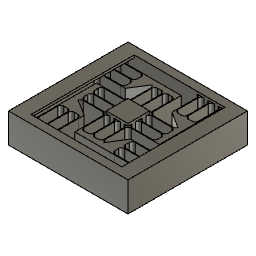
smaller mill draft (Autodesk Fusion 360 design; units mm, degrees)
part number: Configuration 5
Autodesk Fusion 360 part; units mm, degrees
(part 1 of 2)
sketch "Sketch2" plane through (0, 0, 0) normal (0, 0, 1) x (1, 0, 0) in component "xy"
  line L0 (-95, 0) -> (-95, -95)
  line L1 (-95, -95) -> (0, -95)
  line L2 (0, -20) -> (0, 0)
  line L3 (-38, -95) -> (-38, -47)
  line L4 (-78, -95) -> (-78, -47)
  line L5 (0, 0) -> (-20, 0)
  line L6 (-20, 0) -> (-20, -20)
  line L7 (-20, -20) -> (0, -20)
  line L8 (0, -20) -> (0, 0)
  line L9 (-20, -20) -> (-68, -20)
  line L10 (-110, 0) -> (-110, -110)
  line L11 (-110, -110) -> (0, -110)
  line L12 (-68, -24) -> (-38, -43)
  line L13 (-38, -43) -> (-38, -47)
  line L14 (-38, -47) -> (-78, -47)
  line L15 (0, -95) -> (0, -110)
  line L16 (-95, 0) -> (-110, 0)
  line L17 (-95, 0) -> (-110, 0) construction
  line L18 (0, -110) -> (0, -95) construction
  line L19 (0, -20) -> (0, 0) construction
  line L20 (0, 0) -> (-110, 0) construction
  line L21 (-110, 0) -> (-110, -110) construction
  line L22 (-110, -110) -> (0, -110) construction
  line L23 (0, -110) -> (0, 0) construction
  line L24 (-58, -47) -> (-58, -95) construction
  line L25 (-58.9, -71) -> (-57.1, -71) construction
  line L26 (-58.9, -47) -> (-58.9, -95)
  line L27 (-57.1, -95) -> (-57.1, -47)
  line L28 (-39.8, -95) -> (-39.8, -47)
  line L29 (-76.2, -95) -> (-76.2, -47)
  line L30 (-20, -18.2) -> (-68, -18.2)
  line L31 (0, 0) -> (-20, 0)
  line L32 (-190, 0) -> (-210, 0) construction
  line L33 (-20, 0.9) -> (-68, 0.9)
  line L34 (-20, -0.9) -> (-68, -0.9)
  line L35 (-44, -0.9) -> (-44, 0.9) construction
  line L36 (-20, 0.9) -> (-20, 0)
  line L37 (-20, 18.2) -> (-68, 18.2)
  line L38 (-20, 20) -> (-68, 20)
  line L39 (-78, -47) -> (-78, 20)
  line L40 (-78, 20) -> (-68, 20)
  line L41 (-68, 20) -> (-68, -24)
  line L42 (-20, 18.2) -> (-20, 20)
  line L43 (-20, 20) -> (-20, -18.2)
  line L44 (-20, -20) -> (20, -20)
  line L45 (20, -20) -> (20, 20)
  line L46 (20, 20) -> (-20, 20)
  line L47 (-20, 20) -> (-20, -20)
  line L48 (-20, -20) -> (20, 20) construction
  line L49 (20, -20) -> (-20, 20) construction
  point P0 (-44, 0)
  dimension "d47" = 40
  dimension "d48" = 17
  dimension "d52" = 15
  dimension "d56" = 4
  dimension "d57" = 110
  dimension "d60" = -1.8
  dimension "d64" = 40
  dimension "d86" = 10
  dimension "d117" = 4
  constraint vertical L0
  constraint horizontal L1
  constraint vertical L2
  constraint coincident L2.end L5.start
  constraint coincident L1 L3.start
  constraint perpendicular L1 L3
  constraint coincident L1 L4.start
  constraint perpendicular L1 L4
  constraint equal L3 L4
  constraint horizontal L5
  constraint vertical L6
  constraint horizontal L7
  constraint vertical L8
  constraint equal L6 L7
  constraint perpendicular L6 L9
  constraint equal L4 L9
  constraint horizontal L31
  constraint vertical L10
  constraint horizontal L11
  constraint vertical L18
  constraint equal L10 L11
  constraint vertical L13
  constraint horizontal L14
  constraint coincident L4.end L14.end
  constraint coincident L3.end L13.end
  constraint collinear L17 L31
  constraint collinear L18 L19
  constraint horizontal L20
  constraint vertical L21
  constraint horizontal L22
  constraint vertical L23
  constraint equal L0 L1
  constraint midpoint L14 L24.start
  constraint coincident L1 L24.end
  constraint perpendicular L1 L24
  constraint perpendicular L24 L25
  constraint midpoint L24 L25
  constraint coincident L14 L26.start
  constraint coincident L1 L26.end
  constraint perpendicular L1 L26
  constraint coincident L1 L27.start
  constraint coincident L14 L27.end
  constraint perpendicular L14 L27
  constraint coincident L25.start L26
  constraint coincident L25.end L27
  constraint horizontal L33
  constraint parallel L33 L34
  constraint midpoint L34 L35.start
  constraint coincident L33 L35.end
  constraint perpendicular L33 L35
  constraint midpoint L33 L35.end
  constraint equal L33 L34
  constraint coincident L6 L34.start
  constraint midpoint L35 P0
  constraint coincident L20 P0
  constraint symmetric L6.end L20 L38.start
  constraint symmetric L9.end L20 L38.end
  constraint symmetric L20 L30.start L37.start
  constraint symmetric L20 L30.end L37.end
  constraint vertical L39
  constraint horizontal L40
  constraint vertical L41
  constraint coincident L38.end L40.end
  constraint perpendicular L38 L42
  constraint horizontal L44
  constraint perpendicular L44 L45
  constraint parallel L44 L46
  constraint parallel L45 L47
  constraint coincident L48 L2.end
  constraint coincident L49 L2.end
  constraint coincident L33.end L41
  measures "d47" distance of L3 L4
  measures "d48" distance of L0.end L4
  measures "d52" distance of L0 L10
  measures "d56" distance of L9.end L12.start
  measures "d57" distance of L10.start L10.end
  measures "d86" distance of L12.start L39
  measures "d117" distance of L12.end L3.end
extrude "Extrude3" add sketch "Sketch2" along normal mid plane 67.5 contours L2 L5 L8 L31 L36 L42 L43 L44 L45 L46 L47 | L2 L5 L6 L7 L8 L31 L43 L44 L47 makes body 1 in component "xy"
extrude "Extrude2" add sketch "Sketch2" along normal mid plane 67.5 separate body contours L0 L1 L10 L11 L15 L16 | L1 L4 L14 L29 | L12 L13 L14 L39 L40 L41 | L1 L14 L26 L27 | L37 L38 L41 L42 L43 L47 | L1 L3 L14 L28 | L6 L33 L34 L36 L41 L43 L47 | L6 L9 L30 L41 L47 makes body 2 in component "xy"
combine "Combine2" operation add target body 1 tool bodies 2 in component "xy"
fillet "Fillet2" radius 5.558 19 edges at (-20, -18.2, 0) (-20, 0.9, 0) (-20, 18.2, 0) (-20, -0.9, 0) (-68, -18.2, 0) (-68, -20, 0) (-68, 0.9, 0) (-68, -0.9, 0) (-68, 18.2, 0) (-38, -95, 0) (-57.1, -95, 0) (-76.2, -95, 0) (-78, -95, 0) (-39.8, -95, 0) (-58.9, -95, 0) (-76.2, -47, 0) (-57.1, -47, 0) (-39.8, -47, 0) (-58.9, -47, 0) on bodies 1 in component "xy"
pattern_circular "C-Pattern3" count 4 over 360 about axis through (0, 0, 1.75) along (0, 0, 1) of bodies 1 makes body 3 at (110, -73.3333, 11.25) makes body 4 at (73.3333, 110, 11.25) makes body 5 at (-110, 73.3333, 11.25) in component "xy"
combine "Combine3" operation add target body 3 tool bodies 1 5 4 in component "xy"
fillet "Fillet4" radius 6.013 4 edges at (-20, 20, 0) (20, 20, 0) (20, -20, 0) (-20, -20, 0) on bodies 3 in component "xy"
sketch "Sketch3" plane through (0, 0, 33.75) normal (0, 0, 1) x (-1, 0, 0) in component "xy"
  line L0 (-110, -110) -> (110, -110)
  line L1 (110, -110) -> (110, 110)
  line L2 (110, 110) -> (-110, 110)
  line L3 (-110, 110) -> (-110, -110)
  line L4 (-95, -95) -> (-95, 32.442)
  arc A0 (-89.442, 38) -> (-95, 32.442) centre (-89.442, 32.442) ccw
  line L5 (-89.442, 38) -> (-43, 38)
  line L6 (-43, 38) -> (-24, 68)
  arc A1 (-20, 62.6648) -> (-24, 68) centre (-25.558, 62.6648) ccw
  line L7 (-20, 62.6648) -> (-20, 26.013)
  arc A2 (-26.013, 20) -> (-20, 26.013) centre (-26.013, 26.013) ccw
  line L8 (-26.013, 20) -> (-78, 20)
  line L9 (-78, 20) -> (-78, -89.442)
  arc A3 (-83.558, -95) -> (-78, -89.442) centre (-83.558, -89.442) ccw
  line L10 (-83.558, -95) -> (-95, -95)
  line L11 (-20, 12.642) -> (-20, 6.458)
  arc A4 (-25.558, 0.9) -> (-20, 6.458) centre (-25.558, 6.458) ccw
  line L12 (-25.558, 0.9) -> (-62.442, 0.9)
  arc A5 (-68, 6.458) -> (-62.442, 0.9) centre (-62.442, 6.458) ccw
  line L13 (-68, 6.458) -> (-68, 12.642)
  arc A6 (-62.442, 18.2) -> (-68, 12.642) centre (-62.442, 12.642) ccw
  line L14 (-62.442, 18.2) -> (-25.558, 18.2)
  arc A7 (-20, 12.642) -> (-25.558, 18.2) centre (-25.558, 12.642) ccw
  line L15 (-20, -6.458) -> (-20, -12.642)
  arc A8 (-25.558, -18.2) -> (-20, -12.642) centre (-25.558, -12.642) ccw
  line L16 (-25.558, -18.2) -> (-62.442, -18.2)
  arc A9 (-68, -12.642) -> (-62.442, -18.2) centre (-62.442, -12.642) ccw
  line L17 (-68, -12.642) -> (-68, -6.458)
  arc A10 (-62.442, -0.9) -> (-68, -6.458) centre (-62.442, -6.458) ccw
  line L18 (-62.442, -0.9) -> (-25.558, -0.9)
  arc A11 (-20, -6.458) -> (-25.558, -0.9) centre (-25.558, -6.458) ccw
  line L19 (-45.358, -95) -> (-51.542, -95)
  arc A12 (-57.1, -89.442) -> (-51.542, -95) centre (-51.542, -89.442) ccw
  line L20 (-57.1, -89.442) -> (-57.1, -52.558)
  arc A13 (-51.542, -47) -> (-57.1, -52.558) centre (-51.542, -52.558) ccw
  line L21 (-51.542, -47) -> (-45.358, -47)
  arc A14 (-39.8, -52.558) -> (-45.358, -47) centre (-45.358, -52.558) ccw
  line L22 (-39.8, -52.558) -> (-39.8, -89.442)
  arc A15 (-45.358, -95) -> (-39.8, -89.442) centre (-45.358, -89.442) ccw
  line L23 (-70.642, -47) -> (-64.458, -47)
  arc A16 (-58.9, -52.558) -> (-64.458, -47) centre (-64.458, -52.558) ccw
  line L24 (-58.9, -52.558) -> (-58.9, -89.442)
  arc A17 (-64.458, -95) -> (-58.9, -89.442) centre (-64.458, -89.442) ccw
  line L25 (-64.458, -95) -> (-70.642, -95)
  arc A18 (-76.2, -89.442) -> (-70.642, -95) centre (-70.642, -89.442) ccw
  line L26 (-76.2, -89.442) -> (-76.2, -52.558)
  arc A19 (-70.642, -47) -> (-76.2, -52.558) centre (-70.642, -52.558) ccw
  arc A20 (-18.2, 25.558) -> (-12.642, 20) centre (-12.642, 25.558) ccw
  line L27 (-18.2, 25.558) -> (-18.2, 62.442)
  arc A21 (-12.642, 68) -> (-18.2, 62.442) centre (-12.642, 62.442) ccw
  line L28 (-12.642, 68) -> (-6.458, 68)
  arc A22 (-0.9, 62.442) -> (-6.458, 68) centre (-6.458, 62.442) ccw
  line L29 (-0.9, 62.442) -> (-0.9, 25.558)
  arc A23 (-6.458, 20) -> (-0.9, 25.558) centre (-6.458, 25.558) ccw
  line L30 (-6.458, 20) -> (-12.642, 20)
  arc A24 (0.9, 25.558) -> (6.458, 20) centre (6.458, 25.558) ccw
  line L31 (0.9, 25.558) -> (0.9, 62.442)
  arc A25 (6.458, 68) -> (0.9, 62.442) centre (6.458, 62.442) ccw
  line L32 (6.458, 68) -> (12.642, 68)
  arc A26 (18.2, 62.442) -> (12.642, 68) centre (12.642, 62.442) ccw
  line L33 (18.2, 62.442) -> (18.2, 25.558)
  arc A27 (12.642, 20) -> (18.2, 25.558) centre (12.642, 25.558) ccw
  line L34 (12.642, 20) -> (6.458, 20)
  line L35 (20, 26.013) -> (20, 78)
  line L36 (20, 78) -> (-89.442, 78)
  arc A28 (-95, 83.558) -> (-89.442, 78) centre (-89.442, 83.558) ccw
  line L37 (-95, 83.558) -> (-95, 95)
  line L38 (-95, 95) -> (32.442, 95)
  arc A29 (38, 89.442) -> (32.442, 95) centre (32.442, 89.442) ccw
  line L39 (38, 89.442) -> (38, 43)
  line L40 (38, 43) -> (68, 24)
  arc A30 (62.6648, 20) -> (68, 24) centre (62.6648, 25.558) ccw
  line L41 (62.6648, 20) -> (26.013, 20)
  arc A31 (20, 26.013) -> (26.013, 20) centre (26.013, 26.013) ccw
  line L42 (95, -95) -> (-32.442, -95)
  arc A32 (-38, -89.442) -> (-32.442, -95) centre (-32.442, -89.442) ccw
  line L43 (-38, -89.442) -> (-38, -43)
  line L44 (-38, -43) -> (-68, -24)
  arc A33 (-62.6648, -20) -> (-68, -24) centre (-62.6648, -25.558) ccw
  line L45 (-62.6648, -20) -> (-26.013, -20)
  arc A34 (-20, -26.013) -> (-26.013, -20) centre (-26.013, -26.013) ccw
  line L46 (-20, -26.013) -> (-20, -78)
  line L47 (-20, -78) -> (89.442, -78)
  arc A35 (95, -83.558) -> (89.442, -78) centre (89.442, -83.558) ccw
  line L48 (95, -83.558) -> (95, -95)
  arc A36 (25.558, 18.2) -> (20, 12.642) centre (25.558, 12.642) ccw
  line L49 (25.558, 18.2) -> (62.442, 18.2)
  arc A37 (68, 12.642) -> (62.442, 18.2) centre (62.442, 12.642) ccw
  line L50 (68, 12.642) -> (68, 6.458)
  arc A38 (62.442, 0.9) -> (68, 6.458) centre (62.442, 6.458) ccw
  line L51 (62.442, 0.9) -> (25.558, 0.9)
  arc A39 (20, 6.458) -> (25.558, 0.9) centre (25.558, 6.458) ccw
  line L52 (20, 6.458) -> (20, 12.642)
  line L53 (-12.642, -20) -> (-6.458, -20)
  arc A40 (-0.9, -25.558) -> (-6.458, -20) centre (-6.458, -25.558) ccw
  line L54 (-0.9, -25.558) -> (-0.9, -62.442)
  arc A41 (-6.458, -68) -> (-0.9, -62.442) centre (-6.458, -62.442) ccw
  line L55 (-6.458, -68) -> (-12.642, -68)
  arc A42 (-18.2, -62.442) -> (-12.642, -68) centre (-12.642, -62.442) ccw
  line L56 (-18.2, -62.442) -> (-18.2, -25.558)
  arc A43 (-12.642, -20) -> (-18.2, -25.558) centre (-12.642, -25.558) ccw
  arc A44 (25.558, -0.9) -> (20, -6.458) centre (25.558, -6.458) ccw
  line L57 (25.558, -0.9) -> (62.442, -0.9)
  arc A45 (68, -6.458) -> (62.442, -0.9) centre (62.442, -6.458) ccw
  line L58 (68, -6.458) -> (68, -12.642)
  arc A46 (62.442, -18.2) -> (68, -12.642) centre (62.442, -12.642) ccw
  line L59 (62.442, -18.2) -> (25.558, -18.2)
  arc A47 (20, -12.642) -> (25.558, -18.2) centre (25.558, -12.642) ccw
  line L60 (20, -12.642) -> (20, -6.458)
  line L61 (6.458, -20) -> (12.642, -20)
  arc A48 (18.2, -25.558) -> (12.642, -20) centre (12.642, -25.558) ccw
  line L62 (18.2, -25.558) -> (18.2, -62.442)
  arc A49 (12.642, -68) -> (18.2, -62.442) centre (12.642, -62.442) ccw
  line L63 (12.642, -68) -> (6.458, -68)
  arc A50 (0.9, -62.442) -> (6.458, -68) centre (6.458, -62.442) ccw
  line L64 (0.9, -62.442) -> (0.9, -25.558)
  arc A51 (6.458, -20) -> (0.9, -25.558) centre (6.458, -25.558) ccw
  line L65 (-95, 45.358) -> (-95, 51.542)
  arc A52 (-89.442, 57.1) -> (-95, 51.542) centre (-89.442, 51.542) ccw
  line L66 (-89.442, 57.1) -> (-52.558, 57.1)
  arc A53 (-47, 51.542) -> (-52.558, 57.1) centre (-52.558, 51.542) ccw
  line L67 (-47, 51.542) -> (-47, 45.358)
  arc A54 (-52.558, 39.8) -> (-47, 45.358) centre (-52.558, 45.358) ccw
  line L68 (-52.558, 39.8) -> (-89.442, 39.8)
  arc A55 (-95, 45.358) -> (-89.442, 39.8) centre (-89.442, 45.358) ccw
  line L69 (-47, 70.642) -> (-47, 64.458)
  arc A56 (-52.558, 58.9) -> (-47, 64.458) centre (-52.558, 64.458) ccw
  line L70 (-52.558, 58.9) -> (-89.442, 58.9)
  arc A57 (-95, 64.458) -> (-89.442, 58.9) centre (-89.442, 64.458) ccw
  line L71 (-95, 64.458) -> (-95, 70.642)
  arc A58 (-89.442, 76.2) -> (-95, 70.642) centre (-89.442, 70.642) ccw
  line L72 (-89.442, 76.2) -> (-52.558, 76.2)
  arc A59 (-47, 70.642) -> (-52.558, 76.2) centre (-52.558, 70.642) ccw
  line L73 (45.358, 95) -> (51.542, 95)
  arc A60 (57.1, 89.442) -> (51.542, 95) centre (51.542, 89.442) ccw
  line L74 (57.1, 89.442) -> (57.1, 52.558)
  arc A61 (51.542, 47) -> (57.1, 52.558) centre (51.542, 52.558) ccw
  line L75 (51.542, 47) -> (45.358, 47)
  arc A62 (39.8, 52.558) -> (45.358, 47) centre (45.358, 52.558) ccw
  line L76 (39.8, 52.558) -> (39.8, 89.442)
  arc A63 (45.358, 95) -> (39.8, 89.442) centre (45.358, 89.442) ccw
  line L77 (70.642, 47) -> (64.458, 47)
  arc A64 (58.9, 52.558) -> (64.458, 47) centre (64.458, 52.558) ccw
  line L78 (58.9, 52.558) -> (58.9, 89.442)
  arc A65 (64.458, 95) -> (58.9, 89.442) centre (64.458, 89.442) ccw
  line L79 (64.458, 95) -> (70.642, 95)
  arc A66 (76.2, 89.442) -> (70.642, 95) centre (70.642, 89.442) ccw
  line L80 (76.2, 89.442) -> (76.2, 52.558)
  arc A67 (70.642, 47) -> (76.2, 52.558) centre (70.642, 52.558) ccw
  line L81 (47, -70.642) -> (47, -64.458)
  arc A68 (52.558, -58.9) -> (47, -64.458) centre (52.558, -64.458) ccw
  line L82 (52.558, -58.9) -> (89.442, -58.9)
  arc A69 (95, -64.458) -> (89.442, -58.9) centre (89.442, -64.458) ccw
  line L83 (95, -64.458) -> (95, -70.642)
  arc A70 (89.442, -76.2) -> (95, -70.642) centre (89.442, -70.642) ccw
  line L84 (89.442, -76.2) -> (52.558, -76.2)
  arc A71 (47, -70.642) -> (52.558, -76.2) centre (52.558, -70.642) ccw
  line L85 (95, -45.358) -> (95, -51.542)
  arc A72 (89.442, -57.1) -> (95, -51.542) centre (89.442, -51.542) ccw
  line L86 (89.442, -57.1) -> (52.558, -57.1)
  arc A73 (47, -51.542) -> (52.558, -57.1) centre (52.558, -51.542) ccw
  line L87 (47, -51.542) -> (47, -45.358)
  arc A74 (52.558, -39.8) -> (47, -45.358) centre (52.558, -45.358) ccw
  line L88 (52.558, -39.8) -> (89.442, -39.8)
  arc A75 (95, -45.358) -> (89.442, -39.8) centre (89.442, -45.358) ccw
  line L89 (26.013, -20) -> (78, -20)
  line L90 (78, -20) -> (78, 89.442)
  arc A76 (83.558, 95) -> (78, 89.442) centre (83.558, 89.442) ccw
  line L91 (83.558, 95) -> (95, 95)
  line L92 (95, 95) -> (95, -32.442)
  arc A77 (89.442, -38) -> (95, -32.442) centre (89.442, -32.442) ccw
  line L93 (89.442, -38) -> (43, -38)
  line L94 (43, -38) -> (24, -68)
  arc A78 (20, -62.6648) -> (24, -68) centre (25.558, -62.6648) ccw
  line L95 (20, -62.6648) -> (20, -26.013)
  arc A79 (26.013, -20) -> (20, -26.013) centre (26.013, -26.013) ccw
  line L96 (-20, 20) -> (20, 20)
  line L97 (20, 20) -> (20, -20)
  line L98 (20, -20) -> (-20, -20)
  line L99 (-20, -20) -> (-20, 20)
  line L100 (-20, 20) -> (20, -20) construction
  line L101 (20, 20) -> (-20, -20) construction
  line L102 (-95, 95) -> (95, 95)
  line L103 (95, 95) -> (95, -95)
  line L104 (95, -95) -> (-95, -95)
  line L105 (-95, -95) -> (-95, 95)
  line L106 (-95, 95) -> (95, -95) construction
  line L107 (95, 95) -> (-95, -95) construction
  line L108 (-110, 110) -> (110, 110)
  line L109 (110, 110) -> (110, -110)
  line L110 (110, -110) -> (-110, -110)
  line L111 (-110, -110) -> (-110, 110)
  line L112 (-110, 110) -> (110, -110) construction
  line L113 (110, 110) -> (-110, -110) construction
  constraint horizontal L96
  constraint perpendicular L96 L97
  constraint parallel L96 L98
  constraint parallel L97 L99
  constraint coincident L100 origin
  constraint coincident L101 origin
  constraint horizontal L102
  constraint perpendicular L102 L103
  constraint parallel L102 L104
  constraint parallel L103 L105
  constraint coincident L106 origin
  constraint coincident L107 origin
  constraint coincident L37.end L38.start
  constraint horizontal L108
  constraint perpendicular L108 L109
  constraint parallel L108 L110
  constraint parallel L109 L111
  constraint coincident L112 origin
  constraint coincident L113 origin
  constraint coincident L2.end L3.start
extrude "Extrude4" add sketch "Sketch3" along normal blind 1 contours L0 L1 L2 L3 L108 L109 L110 L111 | L11 L15 L30 L34 L52 L53 L60 L61 L96 L97 L98 L99 bodies 3 in component "xy"
sketch "Sketch2 (1)" plane through (0, 0, 0) normal (0, 0, 1) x (1, 0, 0) in component "xy"
copy_body "Body->Comp1" bodies 3 removing the originals makes body 6 in component "main xy flex"
sketch "Sketch3 (2)" plane through (0, 0, 33.75) normal (0, 0, 1) x (-1, 0, 0)
  line L0 (20, 20) -> (20, 12.642)
  arc A0 (25.558, 18.2) -> (20, 12.642) centre (25.558, 12.642) ccw
  line L1 (25.558, 18.2) -> (62.442, 18.2)
  arc A1 (68, 12.642) -> (62.442, 18.2) centre (62.442, 12.642) ccw
  line L2 (68, 12.642) -> (68, 6.458)
  arc A2 (62.442, 0.9) -> (68, 6.458) centre (62.442, 6.458) ccw
  line L3 (62.442, 0.9) -> (25.558, 0.9)
  arc A3 (20, 6.458) -> (25.558, 0.9) centre (25.558, 6.458) ccw
  line L4 (20, 6.458) -> (20, -6.458)
  arc A4 (25.558, -0.9) -> (20, -6.458) centre (25.558, -6.458) ccw
  line L5 (25.558, -0.9) -> (62.442, -0.9)
  arc A5 (68, -6.458) -> (62.442, -0.9) centre (62.442, -6.458) ccw
  line L6 (68, -6.458) -> (68, -12.642)
  arc A6 (62.442, -18.2) -> (68, -12.642) centre (62.442, -12.642) ccw
  line L7 (62.442, -18.2) -> (25.558, -18.2)
  arc A7 (20, -12.642) -> (25.558, -18.2) centre (25.558, -12.642) ccw
  line L8 (20, -12.642) -> (20, -20)
  line L9 (20, -20) -> (12.642, -20)
  arc A8 (18.2, -25.558) -> (12.642, -20) centre (12.642, -25.558) ccw
  line L10 (18.2, -25.558) -> (18.2, -62.442)
  arc A9 (12.642, -68) -> (18.2, -62.442) centre (12.642, -62.442) ccw
  line L11 (12.642, -68) -> (6.458, -68)
  arc A10 (0.9, -62.442) -> (6.458, -68) centre (6.458, -62.442) ccw
  line L12 (0.9, -62.442) -> (0.9, -25.558)
  arc A11 (6.458, -20) -> (0.9, -25.558) centre (6.458, -25.558) ccw
  line L13 (6.458, -20) -> (-6.458, -20)
  arc A12 (-0.9, -25.558) -> (-6.458, -20) centre (-6.458, -25.558) ccw
  line L14 (-0.9, -25.558) -> (-0.9, -62.442)
  arc A13 (-6.458, -68) -> (-0.9, -62.442) centre (-6.458, -62.442) ccw
  line L15 (-6.458, -68) -> (-12.642, -68)
  arc A14 (-18.2, -62.442) -> (-12.642, -68) centre (-12.642, -62.442) ccw
  line L16 (-18.2, -62.442) -> (-18.2, -25.558)
  arc A15 (-12.642, -20) -> (-18.2, -25.558) centre (-12.642, -25.558) ccw
  line L17 (-12.642, -20) -> (-20, -20)
  line L18 (-20, -20) -> (-20, -12.642)
  arc A16 (-25.558, -18.2) -> (-20, -12.642) centre (-25.558, -12.642) ccw
  line L19 (-25.558, -18.2) -> (-62.442, -18.2)
  arc A17 (-68, -12.642) -> (-62.442, -18.2) centre (-62.442, -12.642) ccw
  line L20 (-68, -12.642) -> (-68, -6.458)
  arc A18 (-62.442, -0.9) -> (-68, -6.458) centre (-62.442, -6.458) ccw
  line L21 (-62.442, -0.9) -> (-25.558, -0.9)
  arc A19 (-20, -6.458) -> (-25.558, -0.9) centre (-25.558, -6.458) ccw
  line L22 (-20, -6.458) -> (-20, 6.458)
  arc A20 (-25.558, 0.9) -> (-20, 6.458) centre (-25.558, 6.458) ccw
  line L23 (-25.558, 0.9) -> (-62.442, 0.9)
  arc A21 (-68, 6.458) -> (-62.442, 0.9) centre (-62.442, 6.458) ccw
  line L24 (-68, 6.458) -> (-68, 12.642)
  arc A22 (-62.442, 18.2) -> (-68, 12.642) centre (-62.442, 12.642) ccw
  line L25 (-62.442, 18.2) -> (-25.558, 18.2)
  arc A23 (-20, 12.642) -> (-25.558, 18.2) centre (-25.558, 12.642) ccw
  line L26 (-20, 12.642) -> (-20, 20)
  line L27 (-20, 20) -> (-12.642, 20)
  arc A24 (-18.2, 25.558) -> (-12.642, 20) centre (-12.642, 25.558) ccw
  line L28 (-18.2, 25.558) -> (-18.2, 62.442)
  arc A25 (-12.642, 68) -> (-18.2, 62.442) centre (-12.642, 62.442) ccw
  line L29 (-12.642, 68) -> (-6.458, 68)
  arc A26 (-0.9, 62.442) -> (-6.458, 68) centre (-6.458, 62.442) ccw
  line L30 (-0.9, 62.442) -> (-0.9, 25.558)
  arc A27 (-6.458, 20) -> (-0.9, 25.558) centre (-6.458, 25.558) ccw
  line L31 (-6.458, 20) -> (6.458, 20)
  arc A28 (0.9, 25.558) -> (6.458, 20) centre (6.458, 25.558) ccw
  line L32 (0.9, 25.558) -> (0.9, 62.442)
  arc A29 (6.458, 68) -> (0.9, 62.442) centre (6.458, 62.442) ccw
  line L33 (6.458, 68) -> (12.642, 68)
  arc A30 (18.2, 62.442) -> (12.642, 68) centre (12.642, 62.442) ccw
  line L34 (18.2, 62.442) -> (18.2, 25.558)
  arc A31 (12.642, 20) -> (18.2, 25.558) centre (12.642, 25.558) ccw
  line L35 (12.642, 20) -> (20, 20)
  line L36 (-95, 83.558) -> (-95, 70.642)
  arc A32 (-89.442, 76.2) -> (-95, 70.642) centre (-89.442, 70.642) ccw
  line L37 (-89.442, 76.2) -> (-52.558, 76.2)
  arc A33 (-47, 70.642) -> (-52.558, 76.2) centre (-52.558, 70.642) ccw
  line L38 (-47, 70.642) -> (-47, 64.458)
  arc A34 (-52.558, 58.9) -> (-47, 64.458) centre (-52.558, 64.458) ccw
  line L39 (-52.558, 58.9) -> (-89.442, 58.9)
  arc A35 (-95, 64.458) -> (-89.442, 58.9) centre (-89.442, 64.458) ccw
  line L40 (-95, 64.458) -> (-95, 51.542)
  arc A36 (-89.442, 57.1) -> (-95, 51.542) centre (-89.442, 51.542) ccw
  line L41 (-89.442, 57.1) -> (-52.558, 57.1)
  arc A37 (-47, 51.542) -> (-52.558, 57.1) centre (-52.558, 51.542) ccw
  line L42 (-47, 51.542) -> (-47, 45.358)
  arc A38 (-52.558, 39.8) -> (-47, 45.358) centre (-52.558, 45.358) ccw
  line L43 (-52.558, 39.8) -> (-89.442, 39.8)
  arc A39 (-95, 45.358) -> (-89.442, 39.8) centre (-89.442, 45.358) ccw
  line L44 (-95, 45.358) -> (-95, 32.442)
  arc A40 (-89.442, 38) -> (-95, 32.442) centre (-89.442, 32.442) ccw
  line L45 (-89.442, 38) -> (-43, 38)
  line L46 (-43, 38) -> (-24, 68)
  arc A41 (-20, 62.6648) -> (-24, 68) centre (-25.558, 62.6648) ccw
  line L47 (-20, 62.6648) -> (-20, 26.013)
  arc A42 (-26.013, 20) -> (-20, 26.013) centre (-26.013, 26.013) ccw
  line L48 (-26.013, 20) -> (-78, 20)
  line L49 (-78, 20) -> (-78, -89.442)
  arc A43 (-83.558, -95) -> (-78, -89.442) centre (-83.558, -89.442) ccw
  line L50 (-83.558, -95) -> (-70.642, -95)
  arc A44 (-76.2, -89.442) -> (-70.642, -95) centre (-70.642, -89.442) ccw
  line L51 (-76.2, -89.442) -> (-76.2, -52.558)
  arc A45 (-70.642, -47) -> (-76.2, -52.558) centre (-70.642, -52.558) ccw
  line L52 (-70.642, -47) -> (-64.458, -47)
  arc A46 (-58.9, -52.558) -> (-64.458, -47) centre (-64.458, -52.558) ccw
  line L53 (-58.9, -52.558) -> (-58.9, -89.442)
  arc A47 (-64.458, -95) -> (-58.9, -89.442) centre (-64.458, -89.442) ccw
  line L54 (-64.458, -95) -> (-51.542, -95)
  arc A48 (-57.1, -89.442) -> (-51.542, -95) centre (-51.542, -89.442) ccw
  line L55 (-57.1, -89.442) -> (-57.1, -52.558)
  arc A49 (-51.542, -47) -> (-57.1, -52.558) centre (-51.542, -52.558) ccw
  line L56 (-51.542, -47) -> (-45.358, -47)
  arc A50 (-39.8, -52.558) -> (-45.358, -47) centre (-45.358, -52.558) ccw
  line L57 (-39.8, -52.558) -> (-39.8, -89.442)
  arc A51 (-45.358, -95) -> (-39.8, -89.442) centre (-45.358, -89.442) ccw
  line L58 (-45.358, -95) -> (-32.442, -95)
  arc A52 (-38, -89.442) -> (-32.442, -95) centre (-32.442, -89.442) ccw
  line L59 (-38, -89.442) -> (-38, -43)
  line L60 (-38, -43) -> (-68, -24)
  arc A53 (-62.6648, -20) -> (-68, -24) centre (-62.6648, -25.558) ccw
  line L61 (-62.6648, -20) -> (-26.013, -20)
  arc A54 (-20, -26.013) -> (-26.013, -20) centre (-26.013, -26.013) ccw
  line L62 (-20, -26.013) -> (-20, -78)
  line L63 (-20, -78) -> (89.442, -78)
  arc A55 (95, -83.558) -> (89.442, -78) centre (89.442, -83.558) ccw
  line L64 (95, -83.558) -> (95, -70.642)
  arc A56 (89.442, -76.2) -> (95, -70.642) centre (89.442, -70.642) ccw
  line L65 (89.442, -76.2) -> (52.558, -76.2)
  arc A57 (47, -70.642) -> (52.558, -76.2) centre (52.558, -70.642) ccw
  line L66 (47, -70.642) -> (47, -64.458)
  arc A58 (52.558, -58.9) -> (47, -64.458) centre (52.558, -64.458) ccw
  line L67 (52.558, -58.9) -> (89.442, -58.9)
  arc A59 (95, -64.458) -> (89.442, -58.9) centre (89.442, -64.458) ccw
  line L68 (95, -64.458) -> (95, -51.542)
  arc A60 (89.442, -57.1) -> (95, -51.542) centre (89.442, -51.542) ccw
  line L69 (89.442, -57.1) -> (52.558, -57.1)
  arc A61 (47, -51.542) -> (52.558, -57.1) centre (52.558, -51.542) ccw
  line L70 (47, -51.542) -> (47, -45.358)
  arc A62 (52.558, -39.8) -> (47, -45.358) centre (52.558, -45.358) ccw
  line L71 (52.558, -39.8) -> (89.442, -39.8)
  arc A63 (95, -45.358) -> (89.442, -39.8) centre (89.442, -45.358) ccw
  line L72 (95, -45.358) -> (95, -32.442)
  arc A64 (89.442, -38) -> (95, -32.442) centre (89.442, -32.442) ccw
  line L73 (89.442, -38) -> (43, -38)
  line L74 (43, -38) -> (24, -68)
  arc A65 (20, -62.6648) -> (24, -68) centre (25.558, -62.6648) ccw
  line L75 (20, -62.6648) -> (20, -26.013)
  arc A66 (26.013, -20) -> (20, -26.013) centre (26.013, -26.013) ccw
  line L76 (26.013, -20) -> (78, -20)
  line L77 (78, -20) -> (78, 89.442)
  arc A67 (83.558, 95) -> (78, 89.442) centre (83.558, 89.442) ccw
  line L78 (83.558, 95) -> (70.642, 95)
  arc A68 (76.2, 89.442) -> (70.642, 95) centre (70.642, 89.442) ccw
  line L79 (76.2, 89.442) -> (76.2, 52.558)
  arc A69 (70.642, 47) -> (76.2, 52.558) centre (70.642, 52.558) ccw
  line L80 (70.642, 47) -> (64.458, 47)
  arc A70 (58.9, 52.558) -> (64.458, 47) centre (64.458, 52.558) ccw
  line L81 (58.9, 52.558) -> (58.9, 89.442)
  arc A71 (64.458, 95) -> (58.9, 89.442) centre (64.458, 89.442) ccw
  line L82 (64.458, 95) -> (51.542, 95)
  arc A72 (57.1, 89.442) -> (51.542, 95) centre (51.542, 89.442) ccw
  line L83 (57.1, 89.442) -> (57.1, 52.558)
  arc A73 (51.542, 47) -> (57.1, 52.558) centre (51.542, 52.558) ccw
  line L84 (51.542, 47) -> (45.358, 47)
  arc A74 (39.8, 52.558) -> (45.358, 47) centre (45.358, 52.558) ccw
  line L85 (39.8, 52.558) -> (39.8, 89.442)
  arc A75 (45.358, 95) -> (39.8, 89.442) centre (45.358, 89.442) ccw
  line L86 (45.358, 95) -> (32.442, 95)
  arc A76 (38, 89.442) -> (32.442, 95) centre (32.442, 89.442) ccw
  line L87 (38, 89.442) -> (38, 43)
  line L88 (38, 43) -> (68, 24)
  arc A77 (62.6648, 20) -> (68, 24) centre (62.6648, 25.558) ccw
  line L89 (62.6648, 20) -> (26.013, 20)
  arc A78 (20, 26.013) -> (26.013, 20) centre (26.013, 26.013) ccw
  line L90 (20, 26.013) -> (20, 78)
  line L91 (20, 78) -> (-89.442, 78)
  arc A79 (-95, 83.558) -> (-89.442, 78) centre (-89.442, 83.558) ccw
  arc A80 (20, 26.013) -> (26.013, 20) centre (26.013, 26.013) ccw
  line L92 (26.013, 20) -> (62.6648, 20)
  arc A81 (-26.013, 20) -> (-20, 26.013) centre (-26.013, 26.013) ccw
  line L93 (-78, 20) -> (-26.013, 20)
  arc A82 (-20, -26.013) -> (-26.013, -20) centre (-26.013, -26.013) ccw
  line L94 (-26.013, -20) -> (-62.6648, -20)
  arc A83 (26.013, -20) -> (20, -26.013) centre (26.013, -26.013) ccw
  line L95 (20, -26.013) -> (20, -62.6648)
  arc A84 (-58.9, -52.558) -> (-64.458, -47) centre (-64.458, -52.558) ccw
  line L96 (-58.9, -89.442) -> (-58.9, -52.558)
  arc A85 (-39.8, -52.558) -> (-45.358, -47) centre (-45.358, -52.558) ccw
  line L97 (-39.8, -89.442) -> (-39.8, -52.558)
  arc A86 (-51.542, -47) -> (-57.1, -52.558) centre (-51.542, -52.558) ccw
  line L98 (-45.358, -47) -> (-51.542, -47)
  arc A87 (-70.642, -47) -> (-76.2, -52.558) centre (-70.642, -52.558) ccw
  line L99 (-76.2, -52.558) -> (-76.2, -89.442)
  arc A88 (-64.458, -95) -> (-58.9, -89.442) centre (-64.458, -89.442) ccw
  arc A89 (-45.358, -95) -> (-39.8, -89.442) centre (-45.358, -89.442) ccw
  arc A90 (-83.558, -95) -> (-78, -89.442) centre (-83.558, -89.442) ccw
  line L100 (-95, -95) -> (-83.558, -95)
  line L101 (-32.442, -95) -> (95, -95)
  line L102 (-51.542, -95) -> (-45.358, -95)
  line L103 (-70.642, -95) -> (-64.458, -95)
  arc A91 (-76.2, -89.442) -> (-70.642, -95) centre (-70.642, -89.442) ccw
  arc A92 (-57.1, -89.442) -> (-51.542, -95) centre (-51.542, -89.442) ccw
  line L104 (-57.1, -52.558) -> (-57.1, -89.442)
  arc A93 (-38, -89.442) -> (-32.442, -95) centre (-32.442, -89.442) ccw
  line L105 (-38, -43) -> (-38, -89.442)
  arc A94 (-62.442, 18.2) -> (-68, 12.642) centre (-62.442, 12.642) ccw
  line L106 (-25.558, 18.2) -> (-62.442, 18.2)
  arc A95 (-62.442, -0.9) -> (-68, -6.458) centre (-62.442, -6.458) ccw
  line L107 (-25.558, -0.9) -> (-62.442, -0.9)
  arc A96 (-68, 6.458) -> (-62.442, 0.9) centre (-62.442, 6.458) ccw
  line L108 (-68, 12.642) -> (-68, 6.458)
  arc A97 (-62.6648, -20) -> (-68, -24) centre (-62.6648, -25.558) ccw
  arc A98 (-68, -12.642) -> (-62.442, -18.2) centre (-62.442, -12.642) ccw
  line L109 (-68, -6.458) -> (-68, -12.642)
  arc A99 (-20, -6.458) -> (-25.558, -0.9) centre (-25.558, -6.458) ccw
  arc A100 (-20, 12.642) -> (-25.558, 18.2) centre (-25.558, 12.642) ccw
  arc A101 (-25.558, 0.9) -> (-20, 6.458) centre (-25.558, 6.458) ccw
  line L110 (-62.442, 0.9) -> (-25.558, 0.9)
  arc A102 (-25.558, -18.2) -> (-20, -12.642) centre (-25.558, -12.642) ccw
  line L111 (-62.442, -18.2) -> (-25.558, -18.2)
  line L112 (-64.458, -47) -> (-70.642, -47)
  line L113 (-78, -89.442) -> (-78, 20)
  line L114 (-68, -24) -> (-38, -43)
  line L115 (-20, -78) -> (-20, -26.013)
  line L116 (-20, 6.458) -> (-20, 12.642)
  line L117 (-20, -12.642) -> (-20, -6.458)
  line L118 (-20, 26.013) -> (-20, 62.6648)
  arc A103 (52.558, -58.9) -> (47, -64.458) centre (52.558, -64.458) ccw
  line L119 (89.442, -58.9) -> (52.558, -58.9)
  arc A104 (52.558, -39.8) -> (47, -45.358) centre (52.558, -45.358) ccw
  line L120 (89.442, -39.8) -> (52.558, -39.8)
  arc A105 (47, -51.542) -> (52.558, -57.1) centre (52.558, -51.542) ccw
  line L121 (47, -45.358) -> (47, -51.542)
  arc A106 (47, -70.642) -> (52.558, -76.2) centre (52.558, -70.642) ccw
  line L122 (52.558, -76.2) -> (89.442, -76.2)
  arc A107 (95, -64.458) -> (89.442, -58.9) centre (89.442, -64.458) ccw
  arc A108 (95, -45.358) -> (89.442, -39.8) centre (89.442, -45.358) ccw
  arc A109 (95, -83.558) -> (89.442, -78) centre (89.442, -83.558) ccw
  arc A110 (89.442, -76.2) -> (95, -70.642) centre (89.442, -70.642) ccw
  arc A111 (89.442, -57.1) -> (95, -51.542) centre (89.442, -51.542) ccw
  line L123 (52.558, -57.1) -> (89.442, -57.1)
  arc A112 (89.442, -38) -> (95, -32.442) centre (89.442, -32.442) ccw
  line L124 (43, -38) -> (89.442, -38)
  arc A113 (-18.2, -62.442) -> (-12.642, -68) centre (-12.642, -62.442) ccw
  line L125 (-18.2, -25.558) -> (-18.2, -62.442)
  arc A114 (0.9, -62.442) -> (6.458, -68) centre (6.458, -62.442) ccw
  line L126 (0.9, -25.558) -> (0.9, -62.442)
  arc A115 (-6.458, -68) -> (-0.9, -62.442) centre (-6.458, -62.442) ccw
  line L127 (-12.642, -68) -> (-6.458, -68)
  arc A116 (20, -62.6648) -> (24, -68) centre (25.558, -62.6648) ccw
  arc A117 (12.642, -68) -> (18.2, -62.442) centre (12.642, -62.442) ccw
  line L128 (6.458, -68) -> (12.642, -68)
  arc A118 (6.458, -20) -> (0.9, -25.558) centre (6.458, -25.558) ccw
  arc A119 (-12.642, -20) -> (-18.2, -25.558) centre (-12.642, -25.558) ccw
  arc A120 (-0.9, -25.558) -> (-6.458, -20) centre (-6.458, -25.558) ccw
  line L129 (-0.9, -62.442) -> (-0.9, -25.558)
  arc A121 (18.2, -25.558) -> (12.642, -20) centre (12.642, -25.558) ccw
  line L130 (18.2, -62.442) -> (18.2, -25.558)
  line L131 (47, -64.458) -> (47, -70.642)
  line L132 (89.442, -78) -> (-20, -78)
  line L133 (24, -68) -> (43, -38)
  line L134 (110, -110) -> (-110, -110)
  line L135 (78, -20) -> (26.013, -20)
  line L136 (12.642, -20) -> (6.458, -20)
  line L137 (-6.458, -20) -> (-12.642, -20)
  arc A122 (58.9, 52.558) -> (64.458, 47) centre (64.458, 52.558) ccw
  line L138 (58.9, 89.442) -> (58.9, 52.558)
  arc A123 (39.8, 52.558) -> (45.358, 47) centre (45.358, 52.558) ccw
  line L139 (39.8, 89.442) -> (39.8, 52.558)
  arc A124 (51.542, 47) -> (57.1, 52.558) centre (51.542, 52.558) ccw
  line L140 (45.358, 47) -> (51.542, 47)
  arc A125 (70.642, 47) -> (76.2, 52.558) centre (70.642, 52.558) ccw
  line L141 (76.2, 52.558) -> (76.2, 89.442)
  arc A126 (64.458, 95) -> (58.9, 89.442) centre (64.458, 89.442) ccw
  arc A127 (45.358, 95) -> (39.8, 89.442) centre (45.358, 89.442) ccw
  arc A128 (83.558, 95) -> (78, 89.442) centre (83.558, 89.442) ccw
  arc A129 (76.2, 89.442) -> (70.642, 95) centre (70.642, 89.442) ccw
  arc A130 (57.1, 89.442) -> (51.542, 95) centre (51.542, 89.442) ccw
  line L142 (57.1, 52.558) -> (57.1, 89.442)
  arc A131 (38, 89.442) -> (32.442, 95) centre (32.442, 89.442) ccw
  line L143 (38, 43) -> (38, 89.442)
  arc A132 (62.442, -18.2) -> (68, -12.642) centre (62.442, -12.642) ccw
  line L144 (25.558, -18.2) -> (62.442, -18.2)
  arc A133 (62.442, 0.9) -> (68, 6.458) centre (62.442, 6.458) ccw
  line L145 (25.558, 0.9) -> (62.442, 0.9)
  arc A134 (68, -6.458) -> (62.442, -0.9) centre (62.442, -6.458) ccw
  line L146 (68, -12.642) -> (68, -6.458)
  arc A135 (62.6648, 20) -> (68, 24) centre (62.6648, 25.558) ccw
  arc A136 (68, 12.642) -> (62.442, 18.2) centre (62.442, 12.642) ccw
  line L147 (68, 6.458) -> (68, 12.642)
  arc A137 (20, 6.458) -> (25.558, 0.9) centre (25.558, 6.458) ccw
  arc A138 (20, -12.642) -> (25.558, -18.2) centre (25.558, -12.642) ccw
  arc A139 (25.558, -0.9) -> (20, -6.458) centre (25.558, -6.458) ccw
  line L148 (62.442, -0.9) -> (25.558, -0.9)
  arc A140 (25.558, 18.2) -> (20, 12.642) centre (25.558, 12.642) ccw
  line L149 (62.442, 18.2) -> (25.558, 18.2)
  line L150 (64.458, 47) -> (70.642, 47)
  line L151 (95, -32.442) -> (95, 95)
  line L152 (95, -51.542) -> (95, -45.358)
  line L153 (95, -70.642) -> (95, -64.458)
  line L154 (95, -95) -> (95, -83.558)
  line L155 (78, 89.442) -> (78, -20)
  line L156 (68, 24) -> (38, 43)
  line L157 (110, 110) -> (110, -110)
  line L158 (20, 78) -> (20, 26.013)
  line L159 (20, 12.642) -> (20, 6.458)
  line L160 (20, -6.458) -> (20, -12.642)
  line L161 (-110, -110) -> (-110, 110)
  line L162 (-110, 110) -> (110, 110)
  line L163 (-95, 32.442) -> (-95, -95)
  arc A141 (-20, 62.6648) -> (-24, 68) centre (-25.558, 62.6648) ccw
  line L164 (-24, 68) -> (-43, 38)
  line L165 (-43, 38) -> (-89.442, 38)
  arc A142 (-89.442, 38) -> (-95, 32.442) centre (-89.442, 32.442) ccw
  line L166 (-12.642, 20) -> (-6.458, 20)
  arc A143 (-6.458, 20) -> (-0.9, 25.558) centre (-6.458, 25.558) ccw
  line L167 (-0.9, 25.558) -> (-0.9, 62.442)
  arc A144 (-0.9, 62.442) -> (-6.458, 68) centre (-6.458, 62.442) ccw
  line L168 (-6.458, 68) -> (-12.642, 68)
  arc A145 (-12.642, 68) -> (-18.2, 62.442) centre (-12.642, 62.442) ccw
  line L169 (-18.2, 62.442) -> (-18.2, 25.558)
  arc A146 (-18.2, 25.558) -> (-12.642, 20) centre (-12.642, 25.558) ccw
  line L170 (6.458, 20) -> (12.642, 20)
  arc A147 (12.642, 20) -> (18.2, 25.558) centre (12.642, 25.558) ccw
  line L171 (18.2, 25.558) -> (18.2, 62.442)
  arc A148 (18.2, 62.442) -> (12.642, 68) centre (12.642, 62.442) ccw
  line L172 (12.642, 68) -> (6.458, 68)
  arc A149 (6.458, 68) -> (0.9, 62.442) centre (6.458, 62.442) ccw
  line L173 (0.9, 62.442) -> (0.9, 25.558)
  arc A150 (0.9, 25.558) -> (6.458, 20) centre (6.458, 25.558) ccw
  line L174 (32.442, 95) -> (-95, 95)
  line L175 (-95, 95) -> (-95, 83.558)
  arc A151 (-95, 83.558) -> (-89.442, 78) centre (-89.442, 83.558) ccw
  line L176 (-89.442, 78) -> (20, 78)
  line L177 (95, 95) -> (83.558, 95)
  line L178 (51.542, 95) -> (45.358, 95)
  line L179 (70.642, 95) -> (64.458, 95)
  line L180 (-47, 64.458) -> (-47, 70.642)
  arc A152 (-47, 70.642) -> (-52.558, 76.2) centre (-52.558, 70.642) ccw
  line L181 (-52.558, 76.2) -> (-89.442, 76.2)
  arc A153 (-89.442, 76.2) -> (-95, 70.642) centre (-89.442, 70.642) ccw
  line L182 (-95, 70.642) -> (-95, 64.458)
  arc A154 (-95, 64.458) -> (-89.442, 58.9) centre (-89.442, 64.458) ccw
  line L183 (-89.442, 58.9) -> (-52.558, 58.9)
  arc A155 (-52.558, 58.9) -> (-47, 64.458) centre (-52.558, 64.458) ccw
  line L184 (-95, 51.542) -> (-95, 45.358)
  arc A156 (-95, 45.358) -> (-89.442, 39.8) centre (-89.442, 45.358) ccw
  line L185 (-89.442, 39.8) -> (-52.558, 39.8)
  arc A157 (-52.558, 39.8) -> (-47, 45.358) centre (-52.558, 45.358) ccw
  line L186 (-47, 45.358) -> (-47, 51.542)
  arc A158 (-47, 51.542) -> (-52.558, 57.1) centre (-52.558, 51.542) ccw
  line L187 (-52.558, 57.1) -> (-89.442, 57.1)
  arc A159 (-89.442, 57.1) -> (-95, 51.542) centre (-89.442, 51.542) ccw
sketch "Sketch2 (2)" plane through (0, 0, 0) normal (1, 0, 0) x (0, 1, 0) in component "scrue mount"
  line L0 (120, -25) -> (120, 25)
  line L1 (120, 25) -> (93.3333, 25)
  line L2 (93.3333, 25) -> (93.3333, -25)
  line L3 (93.3333, -25) -> (120, -25)
  line L4 (-76.3333, 25) -> (-76.3333, -25)
  line L5 (-76.3333, -25) -> (76.3333, -25)
  line L6 (76.3333, -25) -> (76.3333, 25)
  line L7 (76.3333, 25) -> (-76.3333, 25)
  line L8 (-120, 25) -> (-120, -25)
  line L9 (-120, -25) -> (-93.3333, -25)
  line L10 (-93.3333, -25) -> (-93.3333, 25)
  line L11 (-93.3333, 25) -> (-120, 25)
  line L12 (20, 0) -> (-18.75, 0)
  line L13 (0, 0) -> (0, -171.5306)
  line L14 (0, -35) -> (28.2843, -35)
  line L15 (28.2843, -35) -> (65, -55)
  line L16 (65, -55) -> (0, -55)
  point P0 (-20, 0)
  point P1 (20, 0)
  dimension "scrue_top_stage" = 130
  dimension "d92" = 56.5685
  dimension "d93" = 30
  dimension "d94" = 10
  constraint coincident L13.start origin
  constraint perpendicular L12 L13
  constraint coincident L13 L14.start
  constraint perpendicular L13 L14
  constraint coincident L13 L16.end
  constraint perpendicular L13 L16
  measures "d93" distance of L5 L16
  measures "d94" distance of L5 L14
sketch "Sketch3 (3)" plane through (0, 0, -10) normal (0, 0, -1) x (1, 0, 0) in component "scrue mount"
  line L0 (110, -110) -> (110, 110)
  line L1 (110, 110) -> (-110, 110)
  line L2 (20, -78) -> (20, -26.013)
  line L3 (95, 32.442) -> (95, -95)
  arc A0 (24, 68) -> (20, 62.6648) centre (25.558, 62.6648) ccw
  line L4 (24, 68) -> (43, 38)
  line L5 (43, 38) -> (89.442, 38)
  arc A1 (95, 32.442) -> (89.442, 38) centre (89.442, 32.442) ccw
  arc A2 (6.183, 68) -> (0.625, 62.442) centre (6.183, 62.442) ccw
  arc A3 (-13.192, 68) -> (-18.75, 62.442) centre (-13.192, 62.442) ccw
  line L6 (47, 64.183) -> (47, 71.192)
  arc A4 (89.442, 58.625) -> (95, 64.183) centre (89.442, 64.183) ccw
  arc A5 (89.442, 39.25) -> (95, 44.808) centre (89.442, 44.808) ccw
  line L7 (47, 44.808) -> (47, 51.817)
  line L8 (-32.442, 95) -> (95, 95)
  arc A6 (89.442, 78) -> (95, 83.558) centre (89.442, 83.558) ccw
  line L9 (89.442, 78) -> (-20, 78)
  line L10 (-20, 78) -> (-20, 26.013)
  line L11 (-20, 20) -> (20, 20)
  line L12 (20, 20) -> (20, -20)
  line L13 (20, -20) -> (-20, -20)
  line L14 (-20, -20) -> (-20, 20)
  line L15 (-20, 20) -> (20, -20) construction
  line L16 (20, 20) -> (-20, -20) construction
  line L17 (32.442, -95) -> (-95, -95)
  line L18 (-95, -95) -> (-95, -83.558)
  arc A7 (-89.442, -78) -> (-95, -83.558) centre (-89.442, -83.558) ccw
  line L19 (-89.442, -78) -> (20, -78)
  arc A8 (26.013, -20) -> (20, -26.013) centre (26.013, -26.013) ccw
  line L20 (26.013, -20) -> (62.6648, -20)
  arc A9 (68, -24) -> (62.6648, -20) centre (62.6648, -25.558) ccw
  line L21 (68, -24) -> (38, -43)
  line L22 (38, -43) -> (38, -89.442)
  arc A10 (32.442, -95) -> (38, -89.442) centre (32.442, -89.442) ccw
  line L23 (-110, -110) -> (110, -110)
  line L24 (-110, 110) -> (-110, -110)
  line L25 (95, -95) -> (83.558, -95)
  arc A11 (78, -89.442) -> (83.558, -95) centre (83.558, -89.442) ccw
  line L26 (78, -89.442) -> (78, 20)
  line L27 (78, 20) -> (26.013, 20)
  arc A12 (20, 26.013) -> (26.013, 20) centre (26.013, 26.013) ccw
  line L28 (20, 26.013) -> (20, 62.6648)
  arc A13 (25.558, 18.75) -> (20, 13.192) centre (25.558, 13.192) ccw
  line L29 (25.558, 18.75) -> (62.442, 18.75)
  arc A14 (68, 13.192) -> (62.442, 18.75) centre (62.442, 13.192) ccw
  line L30 (68, 13.192) -> (68, 6.183)
  arc A15 (62.442, 0.625) -> (68, 6.183) centre (62.442, 6.183) ccw
  line L31 (62.442, 0.625) -> (25.558, 0.625)
  arc A16 (20, 6.183) -> (25.558, 0.625) centre (25.558, 6.183) ccw
  line L32 (20, 6.183) -> (20, 13.192)
  line L33 (51.817, -95) -> (44.808, -95)
  arc A17 (39.25, -89.442) -> (44.808, -95) centre (44.808, -89.442) ccw
  line L34 (39.25, -89.442) -> (39.25, -52.558)
  arc A18 (44.808, -47) -> (39.25, -52.558) centre (44.808, -52.558) ccw
  line L35 (44.808, -47) -> (51.817, -47)
  arc A19 (57.375, -52.558) -> (51.817, -47) centre (51.817, -52.558) ccw
  line L36 (57.375, -52.558) -> (57.375, -89.442)
  arc A20 (51.817, -95) -> (57.375, -89.442) centre (51.817, -89.442) ccw
  line L37 (64.183, -47) -> (71.192, -47)
  arc A21 (76.75, -52.558) -> (71.192, -47) centre (71.192, -52.558) ccw
  line L38 (76.75, -52.558) -> (76.75, -89.442)
  arc A22 (71.192, -95) -> (76.75, -89.442) centre (71.192, -89.442) ccw
  line L39 (71.192, -95) -> (64.183, -95)
  arc A23 (58.625, -89.442) -> (64.183, -95) centre (64.183, -89.442) ccw
  line L40 (58.625, -89.442) -> (58.625, -52.558)
  arc A24 (64.183, -47) -> (58.625, -52.558) centre (64.183, -52.558) ccw
  arc A25 (25.558, -0.625) -> (20, -6.183) centre (25.558, -6.183) ccw
  line L41 (25.558, -0.625) -> (62.442, -0.625)
  arc A26 (68, -6.183) -> (62.442, -0.625) centre (62.442, -6.183) ccw
  line L42 (68, -6.183) -> (68, -13.192)
  arc A27 (62.442, -18.75) -> (68, -13.192) centre (62.442, -13.192) ccw
  line L43 (62.442, -18.75) -> (25.558, -18.75)
  arc A28 (20, -13.192) -> (25.558, -18.75) centre (25.558, -13.192) ccw
  line L44 (20, -13.192) -> (20, -6.183)
  line L45 (13.192, 20) -> (6.183, 20)
  arc A29 (0.625, 25.558) -> (6.183, 20) centre (6.183, 25.558) ccw
  line L46 (0.625, 25.558) -> (0.625, 62.442)
  line L47 (6.183, 68) -> (13.192, 68)
  arc A30 (18.75, 62.442) -> (13.192, 68) centre (13.192, 62.442) ccw
  line L48 (18.75, 62.442) -> (18.75, 25.558)
  arc A31 (13.192, 20) -> (18.75, 25.558) centre (13.192, 25.558) ccw
  line L49 (-6.183, 20) -> (-13.192, 20)
  arc A32 (-18.75, 25.558) -> (-13.192, 20) centre (-13.192, 25.558) ccw
  line L50 (-18.75, 25.558) -> (-18.75, 62.442)
  line L51 (-13.192, 68) -> (-6.183, 68)
  arc A33 (-0.625, 62.442) -> (-6.183, 68) centre (-6.183, 62.442) ccw
  line L52 (-0.625, 62.442) -> (-0.625, 25.558)
  arc A34 (-6.183, 20) -> (-0.625, 25.558) centre (-6.183, 25.558) ccw
  line L53 (-26.013, 20) -> (-62.6648, 20)
  arc A35 (-68, 24) -> (-62.6648, 20) centre (-62.6648, 25.558) ccw
  line L54 (-68, 24) -> (-38, 43)
  line L55 (-38, 43) -> (-38, 89.442)
  arc A36 (-32.442, 95) -> (-38, 89.442) centre (-32.442, 89.442) ccw
  line L56 (95, 95) -> (95, 83.558)
  arc A37 (-26.013, 20) -> (-20, 26.013) centre (-26.013, 26.013) ccw
  arc A38 (18.75, -25.558) -> (13.192, -20) centre (13.192, -25.558) ccw
  line L57 (18.75, -25.558) -> (18.75, -62.442)
  arc A39 (13.192, -68) -> (18.75, -62.442) centre (13.192, -62.442) ccw
  line L58 (13.192, -68) -> (6.183, -68)
  arc A40 (0.625, -62.442) -> (6.183, -68) centre (6.183, -62.442) ccw
  line L59 (0.625, -62.442) -> (0.625, -25.558)
  arc A41 (6.183, -20) -> (0.625, -25.558) centre (6.183, -25.558) ccw
  line L60 (6.183, -20) -> (13.192, -20)
  line L61 (-20, 13.192) -> (-20, 6.183)
  arc A42 (-25.558, 0.625) -> (-20, 6.183) centre (-25.558, 6.183) ccw
  line L62 (-25.558, 0.625) -> (-62.442, 0.625)
  arc A43 (-68, 6.183) -> (-62.442, 0.625) centre (-62.442, 6.183) ccw
  line L63 (-68, 6.183) -> (-68, 13.192)
  arc A44 (-62.442, 18.75) -> (-68, 13.192) centre (-62.442, 13.192) ccw
  line L64 (-62.442, 18.75) -> (-25.558, 18.75)
  arc A45 (-20, 13.192) -> (-25.558, 18.75) centre (-25.558, 13.192) ccw
  arc A46 (-0.625, -25.558) -> (-6.183, -20) centre (-6.183, -25.558) ccw
  line L65 (-0.625, -25.558) -> (-0.625, -62.442)
  arc A47 (-6.183, -68) -> (-0.625, -62.442) centre (-6.183, -62.442) ccw
  line L66 (-6.183, -68) -> (-13.192, -68)
  arc A48 (-18.75, -62.442) -> (-13.192, -68) centre (-13.192, -62.442) ccw
  line L67 (-18.75, -62.442) -> (-18.75, -25.558)
  arc A49 (-13.192, -20) -> (-18.75, -25.558) centre (-13.192, -25.558) ccw
  line L68 (-13.192, -20) -> (-6.183, -20)
  line L69 (-20, -6.183) -> (-20, -13.192)
  arc A50 (-25.558, -18.75) -> (-20, -13.192) centre (-25.558, -13.192) ccw
  line L70 (-25.558, -18.75) -> (-62.442, -18.75)
  arc A51 (-68, -13.192) -> (-62.442, -18.75) centre (-62.442, -13.192) ccw
  line L71 (-68, -13.192) -> (-68, -6.183)
  arc A52 (-62.442, -0.625) -> (-68, -6.183) centre (-62.442, -6.183) ccw
  line L72 (-62.442, -0.625) -> (-25.558, -0.625)
  arc A53 (-20, -6.183) -> (-25.558, -0.625) centre (-25.558, -6.183) ccw
  line L73 (-20, -26.013) -> (-20, -62.6648)
  arc A54 (-24, -68) -> (-20, -62.6648) centre (-25.558, -62.6648) ccw
  line L74 (-24, -68) -> (-43, -38)
  line L75 (-43, -38) -> (-89.442, -38)
  arc A55 (-95, -32.442) -> (-89.442, -38) centre (-89.442, -32.442) ccw
  line L76 (-95, -32.442) -> (-95, 95)
  line L77 (-95, 95) -> (-83.558, 95)
  arc A56 (-78, 89.442) -> (-83.558, 95) centre (-83.558, 89.442) ccw
  line L78 (-78, 89.442) -> (-78, -20)
  line L79 (-78, -20) -> (-26.013, -20)
  arc A57 (-20, -26.013) -> (-26.013, -20) centre (-26.013, -26.013) ccw
  line L80 (-95, -51.817) -> (-95, -44.808)
  arc A58 (-89.442, -39.25) -> (-95, -44.808) centre (-89.442, -44.808) ccw
  line L81 (-89.442, -39.25) -> (-52.558, -39.25)
  arc A59 (-47, -44.808) -> (-52.558, -39.25) centre (-52.558, -44.808) ccw
  line L82 (-47, -44.808) -> (-47, -51.817)
  arc A60 (-52.558, -57.375) -> (-47, -51.817) centre (-52.558, -51.817) ccw
  line L83 (-52.558, -57.375) -> (-89.442, -57.375)
  arc A61 (-95, -51.817) -> (-89.442, -57.375) centre (-89.442, -51.817) ccw
  line L84 (-47, -64.183) -> (-47, -71.192)
  arc A62 (-52.558, -76.75) -> (-47, -71.192) centre (-52.558, -71.192) ccw
  line L85 (-52.558, -76.75) -> (-89.442, -76.75)
  arc A63 (-95, -71.192) -> (-89.442, -76.75) centre (-89.442, -71.192) ccw
  line L86 (-95, -71.192) -> (-95, -64.183)
  arc A64 (-89.442, -58.625) -> (-95, -64.183) centre (-89.442, -64.183) ccw
  line L87 (-89.442, -58.625) -> (-52.558, -58.625)
  arc A65 (-47, -64.183) -> (-52.558, -58.625) centre (-52.558, -64.183) ccw
  line L88 (-51.817, 95) -> (-44.808, 95)
  arc A66 (-39.25, 89.442) -> (-44.808, 95) centre (-44.808, 89.442) ccw
  line L89 (-39.25, 89.442) -> (-39.25, 52.558)
  arc A67 (-44.808, 47) -> (-39.25, 52.558) centre (-44.808, 52.558) ccw
  line L90 (-44.808, 47) -> (-51.817, 47)
  arc A68 (-57.375, 52.558) -> (-51.817, 47) centre (-51.817, 52.558) ccw
  line L91 (-57.375, 52.558) -> (-57.375, 89.442)
  arc A69 (-51.817, 95) -> (-57.375, 89.442) centre (-51.817, 89.442) ccw
  line L92 (-64.183, 47) -> (-71.192, 47)
  arc A70 (-76.75, 52.558) -> (-71.192, 47) centre (-71.192, 52.558) ccw
  line L93 (-76.75, 52.558) -> (-76.75, 89.442)
  arc A71 (-71.192, 95) -> (-76.75, 89.442) centre (-71.192, 89.442) ccw
  line L94 (-71.192, 95) -> (-64.183, 95)
  arc A72 (-58.625, 89.442) -> (-64.183, 95) centre (-64.183, 89.442) ccw
  line L95 (-58.625, 89.442) -> (-58.625, 52.558)
  arc A73 (-64.183, 47) -> (-58.625, 52.558) centre (-64.183, 52.558) ccw
  arc A74 (52.558, 76.75) -> (47, 71.192) centre (52.558, 71.192) ccw
  line L96 (52.558, 76.75) -> (89.442, 76.75)
  arc A75 (95, 71.192) -> (89.442, 76.75) centre (89.442, 71.192) ccw
  line L97 (95, 71.192) -> (95, 64.183)
  line L98 (89.442, 58.625) -> (52.558, 58.625)
  arc A76 (47, 64.183) -> (52.558, 58.625) centre (52.558, 64.183) ccw
  line L99 (95, 51.817) -> (95, 44.808)
  line L100 (89.442, 39.25) -> (52.558, 39.25)
  arc A77 (47, 44.808) -> (52.558, 39.25) centre (52.558, 44.808) ccw
  arc A78 (52.558, 57.375) -> (47, 51.817) centre (52.558, 51.817) ccw
  line L101 (52.558, 57.375) -> (89.442, 57.375)
  arc A79 (95, 51.817) -> (89.442, 57.375) centre (89.442, 51.817) ccw
  dimension "d88" = 40
  constraint horizontal L11
  constraint perpendicular L11 L12
  constraint parallel L11 L13
  constraint parallel L12 L14
  constraint coincident L15 origin
  constraint coincident L16 origin
  constraint equal L11 L14
  measures "d88" distance of L11.start L13.end
revolve "Revolve1" [suppressed] in component "scrue mount"
loft "Loft2" [suppressed] in component "scrue mount"
ref_plane "WorkPlane1" through (0, 0, -255) normal (0, 0, -1) x (-1, 0, 0) in component "rotate"
sketch "Sketch1" plane through (0, 0, -255) normal (0, 0, -1) x (-1, 0, 0) in component "bottem scrue mount"
  circle A0 centre (0, 0) radius 65
  dimension "d96" = 130
  constraint coincident A0.centre origin
  measures "d96" diameter of A0
ref_plane "WorkPlane1" through (0, 0, -285) normal (0, 0, -1) x (-1, 0, 0) in component "stage"